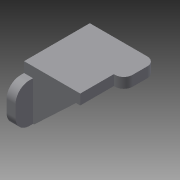
# Autodesk Inventor part: FelixOriginalBase
Saved by Autodesk Inventor 2015 SP1 (Build 190203100, 203)
## iProperties
Created: 2014-12-16
Part Number: FelixOriginalBase
Material: Generic
Document SubType Name: Modeling
Designer: Jack
Density: 1 g/cm^3
Appearance: Default
Author: Jack
Autodesk Inventor part; units mm, degrees
ref_plane "YZ Plane" through (0, 0, 0) normal (1, 0, 0) x (0, 1, 0)
ref_plane "XZ Plane" through (0, 0, 0) normal (0, 1, 0) x (-1, 0, 0)
ref_plane "XY Plane" through (0, 0, 0) normal (0, 0, 1) x (1, 0, 0)
sketch "Sketch1" plane through (0, 0, 0) normal (0, 0, 1) x (1, 0, 0)
  line L0 (0, 0) -> (0, 60.76)
  line L1 (0, 60.76) -> (51.9, 60.76)
  line L2 (51.9, 31.06) -> (51.9, 0)
  line L3 (51.9, 0) -> (0, 0)
  line L4 (51.9, 60.76) -> (61.1, 60.76)
  line L5 (61.1, 60.76) -> (61.1, 31.06)
  line L6 (61.1, 31.06) -> (51.9, 31.06)
  dimension "d0" = 60.76
  dimension "d1" = 51.9
  dimension "d2" = 9.2
  dimension "d3" = 29.7
  constraints: 14 end point, 4 perpendicular, 2 horizontal, 1 vertical, 1 vertical alignment
  measures "d0" distance of L0.start L0.end
  measures "d1" distance of L0.end L1.end
  measures "d2" distance of L1.end L4.end
  measures "d3" distance of L4.end L5.end
extrude "Extrusion1" add sketch "Sketch1" along normal blind 9.5
fillet "Fillet1" radius 8 2 edges at (61.1, 60.76, 4.75) (61.1, 31.06, 4.75)
sketch "Sketch2" plane through (0, 0, 0) normal (0, -1, 0) x (1, 0, 0)
  line L0 (51.9, 0) -> (0, 0) projected
  line L1 (0, -36.5) -> (0, 0)
  line L2 (0, -36.5) -> (9.3, -36.5)
  line L3 (9.3, -36.5) -> (48, 0)
  point P0 (0, 9.5)
  dimension "d7" = 46
  dimension "d8" = 3.9
  dimension "d9" = 9.3
  constraints: 6 end point, 1 horizontal, 1 perpendicular, 1 point on line
  measures "d7" distance of point (0, 9.5) L1.start
  measures "d8" distance of L0.start L3.end
  measures "d9" distance of L1.start L2.end
extrude "Extrusion2" add sketch "Sketch2" against normal blind 7.5
sketch "Sketch3" plane through (0, 60.76, 9.5) normal (0, 1, 0) x (1, 0, 0)
  line L0 (0, 46) -> (0, 9.5) projected
  line L1 (48, 9.5) -> (0, 9.5) projected
  line L2 (48, 9.5) -> (9.3, 46) projected
  line L3 (9.3, 46) -> (0, 46) projected
extrude "Extrusion3" add sketch "Sketch3" against normal blind 10.3
sketch "Sketch4" plane through (0, 0, 9.5) normal (-1, 0, 0) x (0, 0, 1)
  line L0 (-46, 60.76) -> (0, 60.76) projected
  line L1 (-9.5, 7.5) -> (-9.5, 50.46) projected
  line L2 (-46, 0) -> (-46, 7.5) projected
  line L3 (-46, -16.2) -> (-46, 76.96)
  line L4 (-9.5, 76.96) -> (-9.5, -16.2)
  line L5 (-9.5, -16.2) -> (-46, -16.2)
  line L6 (-9.5, 76.96) -> (-46, 76.96)
  point P0 (-9.5, 0)
  dimension "d15" = 93.16
  dimension "d16" = 16.2
  constraints: 8 end point, 2 horizontal, 2 vertical, 1 collinear, 1 point on line
  measures "d15" distance between parallel lines of L6 L5
  measures "d16" distance between parallel lines of L0 L6
extrude "Extrusion4" add sketch "Sketch4" against normal blind 8.3
sketch "Sketch5" plane through (8.3, 0, 9.5) normal (1, 0, 0) x (0, 0, -1)
  line L0 (9.5, 50.46) -> (46, 50.46) projected
  line L1 (9.5, 7.5) -> (9.5, 50.46) projected
  line L2 (46, 7.5) -> (9.5, 7.5) projected
  line L3 (46, 7.5) -> (46, 50.46) projected
  point P0 (9.5, 0)
extrude "Extrusion5" cut sketch "Sketch5" against normal blind 3.3
fillet "Fillet2" radius 12.8 4 edges at (4.15, 76.96, -36.5) (4.15, -16.2, -36.5) (4.15, -16.2, 0) (4.15, 76.96, 0)
body "Solid1"
